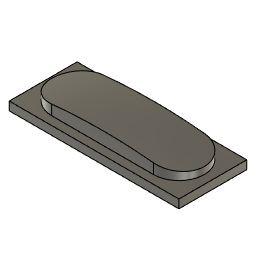
simple-3x-part-cam-challenge (Autodesk Fusion 360 design; units mm, degrees)
Autodesk Fusion 360 part; units mm, degrees
sketch "Sketch1" plane through (0, 0, 0) normal (0, 0, 1) x (1, 0, 0)
  line L0 (63.5, -25.4) -> (-63.5, -25.4)
  line L1 (-63.5, -25.4) -> (-63.5, 25.4)
  line L2 (-63.5, 25.4) -> (63.5, 25.4)
  line L3 (63.5, 25.4) -> (63.5, -25.4)
  line L4 (63.5, -25.4) -> (-63.5, 25.4) construction
  line L5 (-63.5, -25.4) -> (63.5, 25.4) construction
  dimension "d1" = 127
  dimension "d2" = 50.8
  constraint horizontal L0
  constraint perpendicular L0 L1
  constraint parallel L0 L2
  constraint parallel L1 L3
  constraint coincident L4 origin
  constraint coincident L5 origin
  measures "d1" distance of L1.end L2.end
  measures "d2" distance of L0.end L1.end
extrude "Extrude1" add sketch "Sketch1" along normal blind 6.35 makes body 1
sketch "Sketch2" plane through (0, 0, 6.35) normal (0, 0, 1) x (-1, 0, 0)
  line L0 (-63.5, -25.4) -> (63.5, -25.4)
  line L1 (63.5, -25.4) -> (63.5, 25.4)
  line L2 (63.5, 25.4) -> (-63.5, 25.4)
  line L3 (-63.5, 25.4) -> (-63.5, -25.4)
  line L4 (38.1, 19.05) -> (-38.1, 19.05)
  arc A0 (-38.1, 19.05) -> (-38.1, -19.05) centre (-38.1, 0) ccw
  line L5 (-38.1, -19.05) -> (38.1, -19.05)
  arc A1 (38.1, -19.05) -> (38.1, 19.05) centre (38.1, 0) ccw
  line L6 (38.1, 0) -> (-38.1, 0) construction
  dimension "d5" = 38.1
  dimension "d6" = 76.2
  constraint tangent L4 A0
  constraint tangent A0 L5
  constraint parallel L4 L5
  constraint tangent L5 A1
  constraint tangent L4 A1
  constraint perpendicular L1 L6
  constraint midpoint L6 origin
  measures "d5" diameter of A0
  measures "d6" distance of A1.centre A0.centre
extrude "Extrude2" add sketch "Sketch2" along normal blind 12.7 contours L4 A0 L5 A1 bodies 1
sketch "Sketch3" plane through (0, 0, 0) normal (0, 1, 0) x (1, 0, 0)
  line L0 (0, 0) -> (0, -15.875) construction
  arc A0 (-63.5, -10.5461) -> (63.5, -10.5461) centre (0, 365.125) ccw
  dimension "d9" = 15.875
  dimension "d10" = 381
  dimension "d11" = 127
  constraint coincident L0.start origin
  constraint vertical L0
  constraint coincident L0.end A0
  constraint midpoint L0.end A0
  constraint horizontal A0.start A0.end
  measures "d9" distance of L0.start L0.end
  measures "d10" radius of A0
  measures "d11" distance of A0.start A0.end
split "Split1" by curves path "Sketch3" along A0 bodies 1 makes body 2 at (12.7, -6.35, 19.05)
delete_body "RemoveBody1" bodies 2
